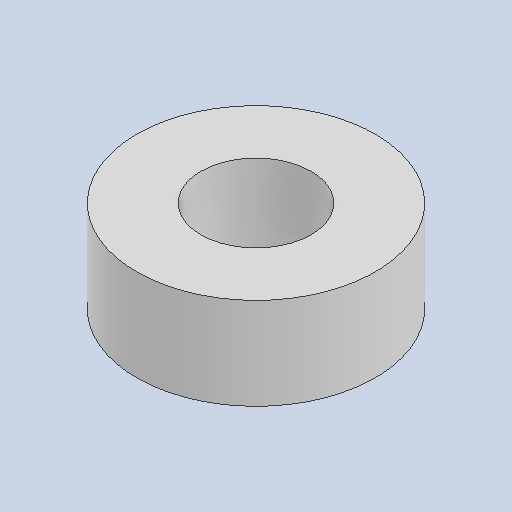
# Autodesk Inventor part: 6x13x5 Bearings
Saved by Autodesk Inventor 2023 (Build 270158000, 158)
## iProperties
Created: 2023-01-18
Part Number: 6x13x5 Bearings
Material: Generic
Document SubType Name: Modeling
Designer: caden
Mass: 0.52229 g
Surface Area: 5.07367 cm^2
Volume: 0.52229 cm^3
Density: 1 g/cm^3
Appearance: Default
Description: https://www.amazon.com/dp/B00Q1AGE7Q?psc=1&pd_rd_i=B00Q1AGE7Q&pd_rd_w=sfk2C&pf_rd_p=887084a2-5c34-4113-a4f8-b7947847c308&pd_rd_wg=HKy52&pf_rd_r=JP22J1XDGZJF1C8B27Y0&pd_rd_r=6cd46cff-9932-47c1-9053-50e1eeb494ea&spLa=ZW5jcnlwdGVkUXVhbGlmaWVyPUEzSk5FQVVPQUdDME9UJmVuY3J5cHRlZElkPUEwOTk0NjM4QjZVNElCMDc4VzhMJmVuY3J5cHRlZEFkSWQ9QTAxODMzMTUzOTdZVUhEQkJKSFMyJndpZGdldE5hbWU9c3BfZGV0YWlsJmFjdGlvbj1jbGlja1JlZGlyZWN0JmRvTm90TG9nQ2xpY2s9dHJ1ZQ%3D%3D&linkCode=sl1&tag=howto045-20&linkId=2c86dbc29cba7eefda55128a0f1644a0&language=en_US&ref_=as_li_ss_tl
Author: caden
Autodesk Inventor part; units mm, degrees
ref_plane "YZ Plane" through (0, 0, 0) normal (1, 0, 0) x (0, 1, 0)
ref_plane "XZ Plane" through (0, 0, 0) normal (0, 1, 0) x (-1, 0, 0)
ref_plane "XY Plane" through (0, 0, 0) normal (0, 0, 1) x (1, 0, 0)
sketch "Sketch1" plane through (0, 0, 0) normal (0, 1, 0) x (-1, 0, 0)
  circle A0 centre (0, 0) radius 6.5
  circle A1 centre (0, 0) radius 3
  dimension "d0" = 13
  dimension "d1" = 6
  constraints: 2 centre point, 2 coincident
  measures "d0" diameter of A0
  measures "d1" diameter of A1
extrude "Extrusion1" add sketch "Sketch1" along normal blind 5
body "Solid1"
